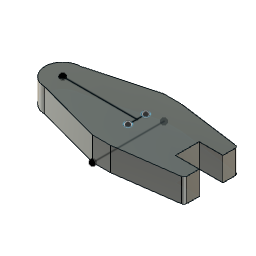
wing_V5L assembly v2 (Autodesk Fusion 360 archive; units mm, degrees)
design "wing_interface_v2"
Autodesk Fusion 360 part; units mm, degrees
sketch "Sketch1" plane through (0, 0, 0) normal (0, 0, 1) x (1, 0, 0)
  line L0 (25, -3) -> (25, 3)
  circle A0 centre (0, 0) radius 0.5
  line L1 (25, 0) -> (21, 0)
  line L2 (21, 0) -> (21, -2)
  line L3 (21, -2) -> (25, -2)
  line L4 (25, -2) -> (25, 0)
  line L5 (25, 0) -> (11, 0)
  line L6 (25, 4.5) -> (25, 0)
  line L7 (11, 0) -> (25, 0)
  line L8 (25, 0) -> (25, -4.5)
  line L9 (25, 0) -> (21, 0)
  line L10 (21, 0) -> (21, 2)
  line L11 (21, 2) -> (25, 2)
  line L12 (25, 2) -> (25, 0)
  line L13 (25, -2) -> (21, -2)
  line L14 (25, -4.5) -> (25, -2)
  line L15 (25, 2) -> (21, 2)
  line L16 (25, 4.5) -> (25, 2)
  line L17 (0, 3) -> (11, 6)
  line L18 (0, -3) -> (11, -6)
  line L19 (11, -6) -> (14, -6)
  line L20 (14, -6) -> (25, -4.5)
  line L21 (11, 6) -> (14, 6)
  line L22 (14, 6) -> (25, 4.5)
  arc A1 (0, 3) -> (0, -3) centre (0, 0) ccw
  dimension "d1" = 6
  dimension "d3" = 1
  constraint coincident A0.centre A1.centre
  constraint vertical L0
  constraint horizontal L1
  constraint vertical L2
  constraint horizontal L3
  constraint vertical L4
  constraint midpoint L0 L1.start
  constraint horizontal L5
  constraint vertical L6
  constraint horizontal L7
  constraint vertical L8
  constraint horizontal L9
  constraint vertical L10
  constraint horizontal L11
  constraint vertical L12
  constraint horizontal L13
  constraint vertical L14
  constraint horizontal L15
  constraint vertical L16
  measures "d1" diameter of A1
  measures "d3" diameter of A0
extrude "Extrude1" add sketch "Sketch1" along normal blind 4 contours L0 L2 L3 L6 L8 L10 L11 L13 L14 L15 L16 L17 L18 L19 L20 L21 L22 A1
fillet "Fillet1" radius 0.5 1 edges at (25, -4.5, 2)
fillet "Fillet2" radius 0.5 1 edges at (25, 4.5, 2)
fillet "Fillet3" radius 0.5 1 edges at (14, 6, 2)
fillet "Fillet4" radius 0.5 1 edges at (11, 6, 2)
fillet "Fillet5" radius 0.5 1 edges at (14, -6, 2)
fillet "Fillet6" radius 0.5 1 edges at (11, -6, 2)
sketch "Sketch2" plane through (0, 0, 0) normal (0, 0, 1) x (1, 0, 0)
sketch "Sketch3" plane through (0, 0, 0) normal (0, 1, 0) x (1, 0, 0)
sketch "Sketch6" plane through (0, 0, 0) normal (0, 0, -1) x (1, 0, 0)
  circle A0 centre (0, 0) radius 0.5
  arc A1 (11.067, 6) -> (10.9354, 5.9824) centre (11.067, 5.5) ccw
  line L0 (10.9354, 5.9824) -> (0, 3)
  arc A2 (0, 3) -> (0, -3) centre (0, 0) ccw
  line L1 (0, -3) -> (10.9354, -5.9824)
  arc A3 (10.9354, -5.9824) -> (11.067, -6) centre (11.067, -5.5) ccw
  line L2 (11.067, -6) -> (13.9661, -6)
  arc A4 (13.9661, -6) -> (14.0336, -5.9954) centre (13.9661, -5.5) ccw
  line L3 (14.0336, -5.9954) -> (24.5676, -4.559)
  arc A5 (24.5676, -4.559) -> (25, -4.0636) centre (24.5, -4.0636) ccw
  line L4 (25, -4.0636) -> (25, -2)
  line L5 (25, -2) -> (21, -2)
  line L6 (21, -2) -> (21, 2)
  line L7 (21, 2) -> (25, 2)
  line L8 (25, 2) -> (25, 4.0636)
  arc A6 (25, 4.0636) -> (24.5676, 4.559) centre (24.5, 4.0636) ccw
  line L9 (24.5676, 4.559) -> (14.0336, 5.9954)
  arc A7 (14.0336, 5.9954) -> (13.9661, 6) centre (13.9661, 5.5) ccw
  line L10 (13.9661, 6) -> (11.067, 6)
  line L11 (11.067, 6) -> (11.067, -6)
  dimension "d22" = 21
  constraint coincident A1.start L10.end
  constraint coincident A3.end L2.start
  measures "d22" distance of A0.centre L6
sketch "Sketch7" plane through (0, 0, 4) normal (0, 0, 1) x (-1, 0, 0)
  arc A0 (-10.9354, 5.9824) -> (-11.067, 6) centre (-11.067, 5.5) ccw
  line L0 (-11.067, 6) -> (-13.9661, 6)
  arc A1 (-13.9661, 6) -> (-14.0336, 5.9954) centre (-13.9661, 5.5) ccw
  line L1 (-14.0336, 5.9954) -> (-24.5676, 4.559)
  arc A2 (-24.5676, 4.559) -> (-25, 4.0636) centre (-24.5, 4.0636) ccw
  line L2 (-25, 4.0636) -> (-25, 2)
  line L3 (-25, 2) -> (-21, 2)
  line L4 (-21, 2) -> (-21, -2)
  line L5 (-21, -2) -> (-25, -2)
  line L6 (-25, -2) -> (-25, -4.0636)
  arc A3 (-25, -4.0636) -> (-24.5676, -4.559) centre (-24.5, -4.0636) ccw
  line L7 (-24.5676, -4.559) -> (-14.0336, -5.9954)
  arc A4 (-14.0336, -5.9954) -> (-13.9661, -6) centre (-13.9661, -5.5) ccw
  line L8 (-13.9661, -6) -> (-11.067, -6)
  arc A5 (-11.067, -6) -> (-10.9354, -5.9824) centre (-11.067, -5.5) ccw
  line L9 (-10.9354, -5.9824) -> (0, -3)
  arc A6 (0, -3) -> (0, 3) centre (0, 0) ccw
  line L10 (0, 3) -> (-10.9354, 5.9824)
  circle A7 centre (0, 0) radius 0.5
  line L11 (0, 0) -> (-12.5, 0)
  line L12 (-12.5, 0) -> (-12.5, -1.5)
  line L13 (-12.5, 0) -> (-12.5, 1.5)
  circle A8 centre (-12.5, -1.5) radius 0.5
  circle A9 centre (-12.5, 1.5) radius 0.5
  dimension "d23" = 12.5
  dimension "d24" = 1
  dimension "d25" = 1
  constraint coincident A6.centre A7.centre
  constraint horizontal L11
  constraint perpendicular L11 L12
  constraint perpendicular L11 L13
  constraint coincident L12.end A8.centre
  constraint coincident L13.end A9.centre
  measures "d23" distance of A6.centre L11.end
  measures "d24" diameter of A8
  measures "d25" diameter of A9
hole "Hole1" at (12.5, 1.5, 4) direction (0, 0, -1) diameter 1 depth 2 tip angle 118
hole "Hole2" at (12.5, -1.5, 4) direction (0, 0, -1) diameter 1 depth 2 tip angle 118
ref_plane "WorkPlane1" through (0, 0, 12) normal (0, 0, 1) x (1, 0, 0)
equation "d25 = mm"

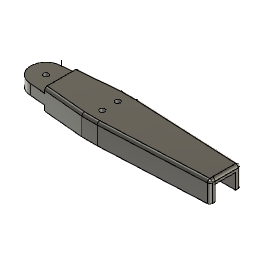
design "wing_interface_V4_p4"
Autodesk Fusion 360 part; units mm, degrees
sketch "Sketch1" plane through (0, 0, 0) normal (0, 0, 1) x (1, 0, 0)
  circle A0 centre (0, 0) radius 3
  line L0 (0, 0) -> (35, 0)
  line L1 (35, 0) -> (35, 3)
  line L2 (14, 4) -> (11, 4)
  line L3 (0, 3) -> (0, 0)
  line L4 (0, 0) -> (35, 0)
  line L5 (35, 0) -> (35, -3)
  line L6 (14, -4) -> (11, -4)
  line L7 (0, -3) -> (0, 0)
  line L8 (35, 0) -> (21, 0)
  line L9 (21, 0) -> (21, 2)
  line L10 (21, 2) -> (35, 2)
  line L11 (35, 2) -> (35, 0)
  line L12 (35, 0) -> (21, 0)
  line L13 (21, 0) -> (21, -2)
  line L14 (21, -2) -> (35, -2)
  line L15 (35, -2) -> (35, 0)
  line L16 (35, 2) -> (35, 3)
  line L17 (35, -2) -> (35, -3)
  line L18 (0, 0) -> (12.5, 0)
  line L19 (12.5, 0) -> (12.5, 1.5)
  line L20 (12.5, 0) -> (12.5, -1.5)
  circle A1 centre (12.5, 1.5) radius 0.5
  circle A2 centre (12.5, -1.5) radius 0.5
  line L21 (0, 3) -> (11, 4)
  line L22 (35, 3) -> (14, 4)
  line L23 (0, -3) -> (11, -4)
  line L24 (35, -3) -> (14, -4)
  dimension "d1" = 6
  dimension "d2" = 35
  dimension "d3" = 14
  dimension "d4" = 14
  dimension "d5" = 12.5
  dimension "d6" = 1.5
  dimension "d7" = 1.5
  dimension "d8" = 1
  dimension "d9" = 1
  constraint coincident A0.centre L0.start
  constraint horizontal L0
  constraint vertical L1
  constraint horizontal L2
  constraint vertical L3
  constraint horizontal L4
  constraint vertical L5
  constraint horizontal L6
  constraint vertical L7
  constraint horizontal L8
  constraint vertical L9
  constraint horizontal L10
  constraint vertical L11
  constraint horizontal L12
  constraint vertical L13
  constraint horizontal L14
  constraint vertical L15
  constraint perpendicular L3 L18
  constraint perpendicular L4 L19
  constraint perpendicular L0 L20
  constraint coincident L19.end A1.centre
  constraint coincident L20.end A2.centre
  constraint coincident A0 L3.start
  constraint coincident A0 L7.start
  measures "d1" diameter of A0
  measures "d2" distance of A0.centre L0.end
  measures "d3" distance of L0.end L8.end
  measures "d4" distance of L0.end L8.end
  measures "d5" distance of A0.centre L18.end
  measures "d6" distance of L18.end L19.end
  measures "d7" distance of L18.end L20.end
  measures "d8" diameter of A1
  measures "d9" diameter of A2
extrude "Extrude1" add sketch "Sketch1" along normal blind 4
sketch "Sketch2" plane through (0, 0, 0) normal (0, 0, -1) x (1, 0, 0)
  circle A0 centre (12.5, -1.5) radius 0.5
  circle A1 centre (12.5, 1.5) radius 0.5
  line L0 (35, -3) -> (35, 2)
  line L1 (35, 2) -> (35, 3)
  line L2 (35, 3) -> (14, 4)
  line L3 (14, 4) -> (11, 4)
  line L4 (11, 4) -> (0, 3)
  arc A2 (0, 3) -> (0, -3) centre (0, 0) ccw
  line L5 (0, -3) -> (11, -4)
  line L6 (11, -4) -> (14, -4)
  line L7 (14, -4) -> (35, -3)
  line L8 (35, 3) -> (35, -3)
  line L9 (35, 0) -> (21, 0)
  line L10 (21, 0) -> (21, 2)
  line L11 (21, 2) -> (35, 2)
  line L12 (35, 2) -> (35, 0)
  line L13 (35, 0) -> (21, 0)
  line L14 (21, 0) -> (21, -2)
  line L15 (21, -2) -> (35, -2)
  line L16 (35, -2) -> (35, 0)
  dimension "d12" = 14
  dimension "d13" = 2
  constraint coincident L1.end L2.start
  constraint coincident L0.start L7.end
  constraint horizontal L9
  constraint vertical L10
  constraint horizontal L11
  constraint vertical L12
  constraint midpoint L8 L9.start
  constraint horizontal L13
  constraint vertical L14
  constraint horizontal L15
  constraint vertical L16
  measures "d12" distance of L9.start L9.end
  measures "d13" distance of L9.start L0.end
extrude "Extrude2" cut sketch "Sketch2" against normal blind 3 contours L0 L8 L9 L13 L14 L15 L16 | L0 L8 L9 L10 L11 L12 L13
sketch "Sketch3" plane through (0, 0, 4) normal (0, 0, 1) x (-1, 0, 0)
  circle A0 centre (-12.5, -1.5) radius 0.5
  circle A1 centre (-12.5, 1.5) radius 0.5
  line L0 (-35, 2) -> (-35, -3)
  line L1 (-35, -3) -> (-14, -4)
  line L2 (-14, -4) -> (-11, -4)
  line L3 (-11, -4) -> (0, -3)
  arc A2 (0, -3) -> (0, 3) centre (0, 0) ccw
  line L4 (0, 3) -> (-11, 4)
  line L5 (-11, 4) -> (-14, 4)
  line L6 (-14, 4) -> (-35, 3)
  line L7 (-35, 3) -> (-35, 2)
  circle A3 centre (0, 0) radius 3
  dimension "d16" = 6
  constraint coincident A2.centre A3.centre
  measures "d16" diameter of A3
extrude "Extrude3" cut sketch "Sketch3" against normal blind 1 contours A2 A3
sketch "Sketch4" plane through (0, 0, 0) normal (0, 0, -1) x (1, 0, 0)
  line L0 (21, 2) -> (35, 2)
  line L1 (35, 2) -> (35, 3)
  line L2 (35, 3) -> (14, 4)
  line L3 (14, 4) -> (11, 4)
  line L4 (11, 4) -> (0, 3)
  arc A0 (0, 3) -> (0, -3) centre (0, 0) ccw
  line L5 (0, -3) -> (11, -4)
  line L6 (11, -4) -> (14, -4)
  line L7 (14, -4) -> (35, -3)
  line L8 (35, -3) -> (35, -2)
  line L9 (35, -2) -> (21, -2)
  line L10 (21, -2) -> (21, 2)
  circle A1 centre (12.5, -1.5) radius 0.5
  circle A2 centre (12.5, 1.5) radius 0.5
  circle A3 centre (0, 0) radius 3
  dimension "d19" = 6
  constraint concentric A0 A3
  measures "d19" diameter of A3
extrude "Extrude4" cut sketch "Sketch4" against normal blind 1 contours A0 A3
sketch "Sketch5" plane through (0, 0, 4) normal (0, 0, 1) x (-1, 0, 0)
  arc A0 (0, 3) -> (0, -3) centre (0, 0) ccw
  line L0 (0, 3) -> (-11, 4)
  line L1 (-11, 4) -> (-14, 4)
  line L2 (-14, 4) -> (-35, 3)
  line L3 (-35, 3) -> (-35, 2)
  line L4 (-35, 2) -> (-35, -3)
  line L5 (-35, -3) -> (-14, -4)
  line L6 (-14, -4) -> (-11, -4)
  line L7 (-11, -4) -> (0, -3)
  circle A1 centre (-12.5, -1.5) radius 0.5
  circle A2 centre (-12.5, 1.5) radius 0.5
  line L8 (-3, 0) -> (-0.0018, 0)
  line L9 (-0.0018, 0) -> (-0.0018, -3.5)
  line L10 (-0.0018, -3.5) -> (-3, -3.5)
  line L11 (-3, -3.5) -> (-3, 0)
  constraint horizontal L8
  constraint vertical L9
  constraint horizontal L10
  constraint vertical L11
  constraint midpoint A0 L8.start
extrude "Extrude5" cut sketch "Sketch5" against normal blind 1 contours A0 L7 L11
sketch "Sketch6" plane through (0, 0, 4) normal (0, 0, 1) x (-1, 0, 0)
  circle A0 centre (-12.5, 1.5) radius 0.5
  circle A1 centre (-12.5, -1.5) radius 0.5
  line L0 (-3, -3.2727) -> (-3, 0)
  arc A2 (0, 3) -> (-3, 0) centre (0, 0) ccw
  line L1 (0, 3) -> (-11, 4)
  line L2 (-11, 4) -> (-14, 4)
  line L3 (-14, 4) -> (-35, 3)
  line L4 (-35, 3) -> (-35, 2)
  line L5 (-35, 2) -> (-35, -3)
  line L6 (-35, -3) -> (-14, -4)
  line L7 (-14, -4) -> (-11, -4)
  line L8 (-11, -4) -> (-3, -3.2727)
  line L9 (-3, 0) -> (0.4438, 0)
  line L10 (0.4438, 0) -> (0.4438, 3.5)
  line L11 (0.4438, 3.5) -> (-3, 3.5)
  line L12 (-3, 3.5) -> (-3, 0)
  constraint horizontal L9
  constraint vertical L10
  constraint horizontal L11
  constraint vertical L12
  constraint coincident L0.end A2.end
extrude "Extrude6" cut sketch "Sketch6" against normal blind 1 contours A2 L1 L12
sketch "Sketch7" plane through (0, 0, 0) normal (0, 0, -1) x (1, 0, 0)
  circle A0 centre (12.5, 1.5) radius 0.5
  circle A1 centre (12.5, -1.5) radius 0.5
  arc A2 (0, -3) -> (0, 3) centre (0, 0) ccw
  line L0 (0, -3) -> (11, -4)
  line L1 (11, -4) -> (14, -4)
  line L2 (14, -4) -> (35, -3)
  line L3 (35, -3) -> (35, -2)
  line L4 (35, -2) -> (21, -2)
  line L5 (21, -2) -> (21, 2)
  line L6 (21, 2) -> (35, 2)
  line L7 (35, 2) -> (35, 3)
  line L8 (35, 3) -> (14, 4)
  line L9 (14, 4) -> (11, 4)
  line L10 (11, 4) -> (0, 3)
  line L11 (3, 0) -> (0, 0)
  line L12 (0, 0) -> (0, 3.3794)
  line L13 (0, 3.3794) -> (3, 3.3794)
  line L14 (3, 3.3794) -> (3, 0)
  constraint horizontal L11
  constraint vertical L12
  constraint horizontal L13
  constraint vertical L14
  constraint midpoint A2 L11.start
extrude "Extrude7" cut sketch "Sketch7" against normal blind 1 contours A2 L10 L14
sketch "Sketch8" plane through (0, 0, 0) normal (0, 0, -1) x (1, 0, 0)
  line L0 (3, 3.2727) -> (3, 0)
  arc A0 (0, -3) -> (3, 0) centre (0, 0) ccw
  line L1 (0, -3) -> (11, -4)
  line L2 (11, -4) -> (14, -4)
  line L3 (14, -4) -> (35, -3)
  line L4 (35, -3) -> (35, -2)
  line L5 (35, -2) -> (21, -2)
  line L6 (21, -2) -> (21, 2)
  line L7 (21, 2) -> (35, 2)
  line L8 (35, 2) -> (35, 3)
  line L9 (35, 3) -> (14, 4)
  line L10 (14, 4) -> (11, 4)
  line L11 (11, 4) -> (3, 3.2727)
  circle A1 centre (12.5, -1.5) radius 0.5
  circle A2 centre (12.5, 1.5) radius 0.5
  line L12 (3, 0) -> (-0.0333, 0)
  line L13 (-0.0333, 0) -> (-0.0333, -3.5)
  line L14 (-0.0333, -3.5) -> (3, -3.5)
  line L15 (3, -3.5) -> (3, 0)
  constraint horizontal L12
  constraint vertical L13
  constraint horizontal L14
  constraint vertical L15
  constraint coincident L0.end A0.end
extrude "Extrude8" cut sketch "Sketch8" against normal blind 1 contours A0 L1 L15
sketch "Sketch9" plane through (0, 0, 3) normal (0, 0, 1) x (-1, 0, 0)
  arc A0 (0, -3) -> (0, 3) centre (0, 0) ccw
  line L0 (0, 3) -> (-3, 3.2727)
  line L1 (-3, 3.2727) -> (-3, -3.2727)
  line L2 (-3, -3.2727) -> (-0.0018, -3.0002)
  line L3 (-0.0018, -3.0002) -> (-0.0018, -3)
  arc A1 (-0.0018, -3) -> (0, -3) centre (0, 0) ccw
  circle A2 centre (0, 0) radius 0.5
  dimension "d30" = 1
  constraint concentric A1 A2
  measures "d30" diameter of A2
hole "Hole1" at (0, 0, 3) direction (0, 0, -1) diameter 1 depth 2 tip angle 180
fillet "Fillet1" radius 0.5 10 edges at (35, -2.5, 4) (35, 0.5, 4) (35, 3, 2) (24.5, 3.5, 4) (35, -3, 2) (24.5, -3.5, 4) (12.5, -4, 4) (7, -3.6364, 4) (7, 3.6364, 4) (12.5, 4, 4)
